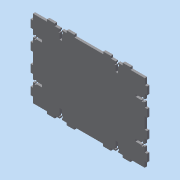
# Autodesk Inventor part: Box Side Panel
Saved by Autodesk Inventor 2013 (Build 170138000, 138)
## iProperties
Created: 2012-12-29
Part Number: Box Side Panel
Material: Generic
Document SubType Name: Modeling
Designer: Administrator
Density: 1 g/cm^3
Author: Administrator
Autodesk Inventor part; units mm, degrees
ref_plane "YZ Plane" through (0, 0, 0) normal (1, 0, 0) x (0, 1, 0)
ref_plane "XZ Plane" through (0, 0, 0) normal (0, 1, 0) x (-1, 0, 0)
ref_plane "XY Plane" through (0, 0, 0) normal (0, 0, 1) x (1, 0, 0)
sketch "Sketch1" plane through (0, 0, 0) normal (0, 0, 1) x (1, 0, 0)
  line L0 (-76.2, 26.9012) -> (-74.2949, 26.9012)
  line L1 (-74.2941, 23.9012) -> (-76.1992, 23.9012)
  line L2 (-74.2949, 28.1566) -> (-71.8949, 28.1566)
  line L3 (-71.8949, 26.9012) -> (-64.316, 26.9012)
  line L4 (-64.316, 26.9012) -> (-64.316, 23.9012)
  line L5 (-64.316, 23.9012) -> (-71.8941, 23.9012)
  line L6 (-71.8941, 23.9012) -> (-71.8941, 22.6512)
  line L7 (-71.8941, 22.6512) -> (-74.2941, 22.6512)
  line L8 (-74.2941, 22.6512) -> (-74.2941, 23.9012)
  line L9 (-71.8949, 28.1566) -> (-71.8949, 26.9012)
  line L10 (-74.2949, 28.1566) -> (-74.2949, 26.9012)
  line L11 (-76.1993, -23.9533) -> (-74.1774, -23.9533)
  line L12 (-74.1774, -26.9533) -> (-76.1993, -26.9533)
  line L13 (-74.1774, -22.7033) -> (-71.7774, -22.7033)
  line L14 (-71.7774, -23.9533) -> (-64.1993, -23.9533)
  line L15 (-64.1993, -23.9533) -> (-64.1993, -26.9533)
  line L16 (-64.1993, -26.9533) -> (-71.7774, -26.9533)
  line L17 (-71.7774, -26.9533) -> (-71.7774, -28.2033)
  line L18 (-71.7774, -28.2033) -> (-74.1774, -28.2033)
  line L19 (-74.1774, -28.2033) -> (-74.1774, -26.9533)
  line L20 (-71.7774, -22.7033) -> (-71.7774, -23.9533)
  line L21 (-74.1774, -22.7033) -> (-74.1774, -23.9533)
  line L22 (68.1553, -28.3527) -> (65.7551, -28.3521)
  line L23 (68.1553, -28.3527) -> (68.1556, -27.1027)
  line L24 (65.7551, -28.3521) -> (65.7555, -27.1021)
  line L25 (65.7555, -27.1021) -> (58.1773, -27.1002)
  line L26 (68.1562, -24.1027) -> (70.1781, -24.1032)
  line L27 (58.1781, -24.1002) -> (65.7562, -24.1021)
  line L28 (65.7562, -24.1021) -> (65.7565, -22.8521)
  line L29 (65.7565, -22.8521) -> (68.1565, -22.8527)
  line L30 (70.1905, -27.1032) -> (68.1556, -27.1027)
  line L31 (58.1773, -27.1002) -> (58.1781, -24.1002)
  line L32 (68.1565, -22.8527) -> (68.1562, -24.1027)
  line L33 (68.3867, 22.4026) -> (65.9867, 22.4026)
  line L34 (68.3867, 22.4026) -> (68.3867, 23.6526)
  line L35 (65.9867, 22.4026) -> (65.9867, 23.6526)
  line L36 (65.9867, 23.6526) -> (58.4085, 23.6526)
  line L37 (68.3863, 26.6526) -> (70.4218, 26.6526)
  line L38 (58.4085, 26.6284) -> (65.9867, 26.6284)
  line L39 (65.9867, 26.6284) -> (65.9867, 27.9026)
  line L40 (65.9867, 27.9026) -> (68.3863, 27.9026)
  line L41 (70.4085, 23.6526) -> (68.3867, 23.6526)
  line L42 (58.4085, 23.6526) -> (58.4085, 26.6284)
  line L43 (68.3863, 27.9026) -> (68.3863, 26.6526)
  line L44 (-38.208, 38.802) -> (-38.2079, 46.5147)
  line L45 (-38.2079, 46.5147) -> (-36.9579, 46.5147)
  line L46 (-36.9579, 46.5147) -> (-36.9579, 48.9147)
  line L47 (-38.2079, 48.9147) -> (-38.2079, 50.802)
  line L48 (-36.9579, 48.9147) -> (-38.2079, 48.9147)
  line L49 (-41.2002, 38.802) -> (-41.2001, 46.5147)
  line L50 (-41.2001, 46.5147) -> (-42.4501, 46.5147)
  line L51 (-42.4501, 48.9147) -> (-41.2001, 48.9147)
  line L52 (-41.2001, 48.9147) -> (-41.2001, 50.802)
  line L53 (-42.4501, 48.9147) -> (-42.4501, 46.5147)
  line L54 (35.2015, 38.8019) -> (35.2015, 46.5146)
  line L55 (35.2015, 46.5146) -> (36.4515, 46.5146)
  line L56 (36.4515, 46.5146) -> (36.4515, 48.9146)
  line L57 (35.2015, 48.9146) -> (35.2015, 50.8019)
  line L58 (36.4515, 48.9146) -> (35.2015, 48.9146)
  line L59 (32.2093, 38.8019) -> (32.2093, 46.5146)
  line L60 (32.2093, 46.5146) -> (30.9593, 46.5146)
  line L61 (30.9593, 48.9146) -> (32.2093, 48.9146)
  line L62 (32.2093, 48.9146) -> (32.2093, 50.8019)
  line L63 (30.9593, 48.9146) -> (30.9593, 46.5146)
  line L64 (-41.197, -48.913) -> (-41.1928, -50.8003)
  line L65 (-38.2102, -38.8003) -> (-38.2102, -46.513)
  line L66 (-38.2102, -46.513) -> (-36.9602, -46.513)
  line L67 (-36.9602, -48.9198) -> (-36.9602, -46.513)
  line L68 (32.1305, -39.158) -> (32.1305, -46.6195)
  line L69 (32.1305, -46.6195) -> (30.8805, -46.6194)
  line L70 (30.8805, -46.6194) -> (30.8805, -49.0194)
  line L71 (30.8805, -49.0194) -> (32.1305, -49.0195)
  line L72 (32.1305, -49.0195) -> (32.1305, -50.8017)
  line L73 (35.1404, -39.158) -> (35.1404, -46.8707)
  line L74 (35.1404, -49.271) -> (35.1404, -50.8078)
  line L75 (35.1404, -46.8707) -> (36.3904, -46.8708)
  line L76 (36.3904, -49.271) -> (36.3904, -46.8708)
  line L77 (36.3904, -49.271) -> (35.1404, -49.271)
  line L78 (-36.9602, -50.8078) -> (-36.9584, -50.8078)
  line L79 (-76.2, 26.9012) -> (-76.2, 33.2012)
  line L80 (-41.2001, 50.802) -> (-47.5001, 50.802)
  line L81 (-47.5001, 50.802) -> (-47.5001, 53.802)
  line L82 (-47.5001, 53.802) -> (-57.5001, 53.8021)
  line L83 (-57.5001, 53.8021) -> (-57.5001, 50.8021)
  line L84 (-57.5001, 50.8021) -> (-76.1999, 50.8022)
  line L85 (-38.2079, 50.802) -> (-31.9079, 50.8019)
  line L86 (-31.9079, 50.8019) -> (-31.9079, 53.8019)
  line L87 (-31.9079, 53.8019) -> (-21.9079, 53.8019)
  line L88 (-21.9079, 53.8019) -> (-21.9079, 50.8019)
  line L89 (-21.9079, 50.8019) -> (15.9093, 50.8019)
  line L90 (32.2093, 50.8019) -> (25.9093, 50.8019)
  line L91 (25.9093, 50.8019) -> (25.9093, 53.8019)
  line L92 (25.9093, 53.8019) -> (15.9093, 53.8019)
  line L93 (15.9093, 53.8019) -> (15.9093, 50.8019)
  line L94 (35.2015, 50.8019) -> (41.5015, 50.8019)
  line L95 (41.5015, 50.8019) -> (41.5015, 53.8019)
  line L96 (41.5015, 53.8019) -> (51.5015, 53.8019)
  line L97 (51.5015, 53.8019) -> (51.5015, 50.8019)
  line L98 (70.4218, 26.6526) -> (70.4218, 32.9526)
  line L99 (70.4218, 32.9526) -> (73.4218, 32.9526)
  line L100 (73.4218, 32.9526) -> (73.4218, 42.9526)
  line L101 (73.4218, 42.9526) -> (70.4085, 42.9526)
  line L102 (70.4085, 42.9526) -> (70.4085, 50.5478)
  line L103 (70.4085, 23.6526) -> (70.4085, 17.3526)
  line L104 (70.4085, 17.3526) -> (73.4218, 17.3526)
  line L105 (73.4218, 17.3526) -> (73.4218, 7.3526)
  line L106 (73.4218, 7.3526) -> (70.1774, 7.3526)
  line L107 (70.1774, 7.3526) -> (70.1774, -7.8032)
  line L108 (70.1781, -24.1032) -> (70.1781, -17.8032)
  line L109 (70.1781, -17.8032) -> (73.1781, -17.8032)
  line L110 (73.1781, -17.8032) -> (73.1781, -7.8032)
  line L111 (73.1781, -7.8032) -> (70.1774, -7.8032)
  line L112 (70.1905, -27.1032) -> (70.1904, -33.4032)
  line L113 (70.1904, -33.4032) -> (73.1904, -33.4032)
  line L114 (73.1904, -33.4032) -> (73.1904, -43.4032)
  line L115 (73.1904, -43.4032) -> (70.201, -43.4032)
  line L116 (70.201, -43.4032) -> (70.2009, -46.5136)
  line L117 (32.1305, -50.8017) -> (25.8305, -50.8017)
  line L118 (25.8305, -50.8017) -> (25.8305, -53.8017)
  line L119 (25.8305, -53.8017) -> (15.8305, -53.8017)
  line L120 (15.8305, -53.8017) -> (15.8305, -50.8076)
  line L121 (15.8305, -50.8076) -> (-15.402, -50.8075)
  line L122 (-41.197, -48.913) -> (-42.447, -48.913)
  line L123 (-42.447, -48.913) -> (-42.447, -46.513)
  line L124 (-42.447, -46.513) -> (-41.2024, -46.513)
  line L125 (-38.2139, -50.8072) -> (-38.2139, -48.9198)
  line L126 (-38.2139, -48.9198) -> (-36.9602, -48.9198)
  line L127 (-41.2024, -46.513) -> (-41.2024, -38.8003)
  line L128 (-38.2139, -50.8072) -> (-31.9139, -50.8072)
  line L129 (-31.9139, -50.8072) -> (-31.9139, -53.8072)
  line L130 (-31.9139, -53.8072) -> (-21.9139, -53.8073)
  line L131 (-21.9139, -53.8073) -> (-21.9139, -50.8074)
  line L132 (-21.9139, -50.8074) -> (-15.402, -50.8075)
  line L133 (-41.1928, -50.8003) -> (-47.4928, -50.8003)
  line L134 (-47.4928, -50.8003) -> (-47.4928, -53.8003)
  line L135 (-47.4928, -53.8003) -> (-57.4928, -53.8002)
  line L136 (-57.4928, -53.8002) -> (-57.4928, -50.8001)
  line L137 (-57.4928, -50.8001) -> (-76.1994, -50.8)
  line L138 (-76.1993, -26.9533) -> (-76.1993, -33.2533)
  line L139 (-76.1993, -33.2533) -> (-79.1993, -33.2533)
  line L140 (-79.1993, -33.2533) -> (-79.1994, -43.2533)
  line L141 (-79.1994, -43.2533) -> (-76.1993, -43.2533)
  line L142 (-76.1993, -43.2533) -> (-76.1994, -50.8)
  line L143 (-76.1993, -23.9533) -> (-76.1993, -17.6533)
  line L144 (-76.1993, -17.6533) -> (-79.1993, -17.6533)
  line L145 (-79.1993, -17.6533) -> (-79.1992, -7.6533)
  line L146 (-79.1992, -7.6533) -> (-76.1993, -7.6533)
  line L147 (-76.1993, -7.6533) -> (-76.1992, 7.3526)
  line L148 (-76.1992, 23.9012) -> (-76.1992, 17.6012)
  line L149 (-76.1992, 17.6012) -> (-79.1992, 17.6012)
  line L150 (-79.1992, 17.6012) -> (-79.1992, 7.6012)
  line L151 (-79.1992, 7.6012) -> (-76.1992, 7.6012)
  line L152 (-76.1992, 7.6012) -> (-76.1992, 7.3526)
  line L153 (35.1404, -50.8078) -> (41.4404, -50.8079)
  line L154 (41.4404, -50.8079) -> (41.4404, -53.8079)
  line L155 (41.4404, -53.8079) -> (51.4404, -53.8079)
  line L156 (51.4404, -53.8079) -> (51.4404, -50.8079)
  line L157 (51.4404, -50.8079) -> (70.2009, -50.8079)
  line L158 (70.2009, -50.8079) -> (70.2009, -46.5136)
  line L159 (51.5015, 50.8019) -> (70.4085, 50.8018)
  line L160 (70.4085, 50.8018) -> (70.4085, 50.5478)
  line L161 (-38.208, 38.802) -> (-41.2002, 38.802)
  line L162 (32.2093, 38.8019) -> (35.2015, 38.8019)
  line L163 (-41.2024, -38.8003) -> (-38.2102, -38.8003)
  line L164 (32.1305, -39.2699) -> (32.1305, -39.158)
  line L165 (35.1404, -39.158) -> (32.1305, -39.158)
  line L166 (-76.2, 33.2012) -> (-79.2, 33.2012)
  line L167 (-79.2, 33.2012) -> (-79.2, 43.2012)
  line L168 (-79.2, 43.2012) -> (-76.2, 43.2012)
  line L169 (-76.2, 43.2012) -> (-76.1999, 50.8022)
  line L170 (-76.2, 38.8022) -> (-76.2, 38.8024)
  point P0 (0, 0)
  dimension "d39" = 12
  dimension "d40" = 3
  dimension "d41" = 7.5781
  dimension "d42" = 2.4
  dimension "d43" = 2.4
  dimension "d44" = 7.5781
  dimension "d45" = 1.25
  dimension "d46" = 1.25
  dimension "d47" = 2.0219
  dimension "d48" = 2.0219
  dimension "d49" = 2.4
  dimension "d50" = 2.4
  dimension "d77" = 2.4
  dimension "d78" = 2.4
  dimension "d89" = 1.25
  dimension "d90" = 2.4
  dimension "d91" = 1.25
  dimension "d95" = 1.25
  dimension "d96" = 2.4
  dimension "d97" = 1.25
  dimension "d102" = 1.25
  dimension "d105" = 1.25
  dimension "d106" = 2.4
  dimension "d107" = 1.25
  dimension "d112" = 6.3
  dimension "d113" = 3
  dimension "d114" = 10
  dimension "d115" = 6.3
  dimension "d116" = 10
  dimension "d117" = 6.3
  dimension "d118" = 3
  dimension "d119" = 10
  dimension "d120" = 6.3
  dimension "d121" = 10
  dimension "d122" = 6.3
  dimension "d123" = 3
  dimension "d124" = 10
  dimension "d125" = 6.3
  dimension "d126" = 10
  dimension "d127" = 6.3
  dimension "d128" = 3
  dimension "d129" = 10
  dimension "d130" = 6.3
  dimension "d131" = 3
  dimension "d132" = 10
  dimension "d136" = 6.3
  dimension "d137" = 3
  dimension "d138" = 10
  dimension "d139" = 1.25
  dimension "d140" = 2.4
  dimension "d142" = 6.3
  dimension "d143" = 3
  dimension "d144" = 10
  dimension "d145" = 90
  dimension "d146" = 6.3
  dimension "d147" = 3
  dimension "d148" = 10
  dimension "d149" = 6.3
  dimension "d150" = 3
  dimension "d151" = 10
  dimension "d152" = 6.3
  dimension "d153" = 3
  dimension "d154" = 10
  dimension "d155" = 6.3
  constraints: 342 end point, 88 perpendicular, 63 parallel, 8 point on line, 3 collinear
  measures "d39" distance of L14.end L11.start
  measures "d40" distance of L14.end L16.start
  measures "d41" distance of L20.end L14.end
  measures "d42" distance of L13.start L13.end
  measures "d43" distance of L17.end L18.end
  measures "d44" distance of L16.start L16.end
  measures "d45" distance of L13.start L21.end
  measures "d46" distance of L16.end L17.end
  measures "d47" horizontal distance of L13.start L11.start
  measures "d48" horizontal distance of L18.end L12.end
  measures "d49" distance of L16.end L12.start
  measures "d50" distance of L20.end L21.end
  measures "d77" distance between parallel lines of L6 L8
  measures "d78" distance between parallel lines of L9 L10
  measures "d89" distance of L44.end L45.end
  measures "d90" distance of L45.end L46.end
  measures "d91" distance of L49.end L50.end
  measures "d95" distance of L54.end L55.end
  measures "d96" distance of L55.end L56.end
  measures "d97" distance of L59.end L60.end
  measures "d102" distance of L65.end L67.end
  measures "d105" distance of L69.start L69.end
  measures "d106" distance of L69.end L70.end
  measures "d107" distance of L73.end L76.end
  measures "d112" distance of L52.end L80.end
  measures "d113" distance of L80.end L81.end
  measures "d114" distance of L81.end L82.end
  measures "d115" distance of L47.end L85.end
  measures "d116" distance of L86.end L87.end
  measures "d117" distance of L62.end L90.end
  measures "d118" distance of L90.end L91.end
  measures "d119" distance of L91.end L92.end
  measures "d120" distance of L57.end L94.end
  measures "d121" distance of L95.end L96.end
  measures "d122" distance of L37.end L98.end
  measures "d123" distance of L98.end L99.end
  measures "d124" distance of L99.end L100.end
  measures "d125" distance of L41.start L103.end
  measures "d126" distance of L104.end L105.end
  measures "d127" distance of L26.end L108.end
  measures "d128" distance of L108.end L109.end
  measures "d129" distance of L109.end L110.end
  measures "d130" distance of L30.start L112.end
  measures "d131" distance of L112.end L113.end
  measures "d132" distance of L113.end L114.end
  measures "d136" distance of L72.end L117.end
  measures "d137" distance of L117.end L118.end
  measures "d138" distance of L118.end L119.end
  measures "d139" distance of L64.start L122.end
  measures "d140" distance of L122.end L123.end
  measures "d142" distance of L125.start L128.end
  measures "d143" distance of L128.end L129.end
  measures "d144" distance of L129.end L130.end
  measures "d145" angle of L130 L129
  measures "d146" distance of L64.end L133.end
  measures "d147" distance of L133.end L134.end
  measures "d148" distance of L134.end L135.end
  measures "d149" distance of L12.end L138.end
  measures "d150" distance of L138.end L139.end
  measures "d151" distance of L139.end L140.end
  measures "d152" distance of L11.start L143.end
  measures "d153" distance of L143.end L144.end
  measures "d154" distance of L144.end L145.end
  measures "d155" distance of L1.end L148.end
extrude "Extrusion4" add sketch "Sketch1" along normal blind 3
body "Solid4"
